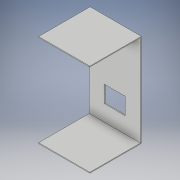
# Autodesk Inventor part: Platinenhalter
Saved by Autodesk Inventor 2017.3 (Build 213256000, 256)
## iProperties
Part Number: Platinenhalter
Material: Generisch
Document SubType Name: Modeling
Designer: Nils
Density: 1 g/cm^3
Appearance: Vorgabe
Author: Nils
Autodesk Inventor part; units mm, degrees
ref_plane "YZ Plane" through (0, 0, 0) normal (1, 0, 0) x (0, 1, 0)
ref_plane "XZ Plane" through (0, 0, 0) normal (0, 1, 0) x (-1, 0, 0)
ref_plane "XY Plane" through (0, 0, 0) normal (0, 0, 1) x (1, 0, 0)
sketch "Skizze1" plane through (0, 0, 0) normal (1, 0, 0) x (0, 1, 0)
  line L0 (-45.75, 82.5) -> (45.75, 82.5)
  line L1 (45.75, 82.5) -> (45.75, -82.5)
  line L2 (45.75, -82.5) -> (-45.75, -82.5)
  line L3 (-45.75, 81) -> (44.25, 81)
  line L4 (44.25, 81) -> (44.25, -81)
  line L5 (44.25, -81) -> (-45.75, -81)
  line L6 (-45.75, -82.5) -> (-45.75, -81)
  line L7 (-45.75, 81) -> (-45.75, 82.5)
  point P0 (0, 0)
  point P1 (0, 82.5)
  point P2 (45.75, 0)
  dimension "d0" = 1.5
  dimension "d1" = 1.5
  dimension "d2" = 1.5
  dimension "d3" = 90
  dimension "d4" = 165
  constraints: 16 end point, 4 parallel, 2 horizontal, 2 midpoint, 2 perpendicular, 2 vertical alignment, 1 horizontal alignment
  measures "d0" distance of L3.start L0.start
  measures "d1" distance of L2.end L5.end
  measures "d2" distance between parallel lines of L1 L4
  measures "d3" distance of L3.start L3.end
  measures "d4" distance of L0.end L1.end
extrude "Extrusion1" add sketch "Skizze1" along normal mid plane 91
sketch "Skizze2" plane through (-45.5, 45.75, 82.5) normal (0, 1, 0) x (1, 0, 0)
  line L0 (64, 105) -> (27, 105)
  line L1 (27, 105) -> (27, 135)
  line L2 (27, 135) -> (64, 135)
  line L3 (64, 135) -> (64, 105)
  line L4 (91, 165) -> (0, 165) projected
  line L5 (91, 165) -> (91, 0) projected
  line L6 (0, 0) -> (0, 165) projected
  point P0 (45.5, 82.5)
  dimension "d7" = 30
  dimension "d8" = 30
  dimension "d9" = 27
  dimension "d10" = 27
  constraints: 8 end point, 2 parallel, 1 horizontal, 1 perpendicular
  measures "d7" distance between parallel lines of L4 L2
  measures "d8" distance of L2.end L0.start
  measures "d9" distance between parallel lines of L3 L5
  measures "d10" distance between parallel lines of L6 L1
extrude "Extrusion2" cut sketch "Skizze2" against normal through all
